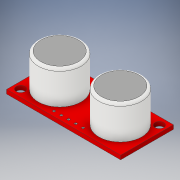
# Autodesk Inventor part: SRF08
Saved by Autodesk Inventor 2018 (Build 220112000, 112)
## iProperties
Created: 2019-03-05
Part Number: SRF08
Material: Generisch
Document SubType Name: Modeling
Designer: RedBots
Density: 1.3582 g/cm^3
Appearance: Vorgabe
Mass: 9 g
Surface Area: 32.6581 cm^2
Volume: 6.62642 cm^3
Author: RedBots
Autodesk Inventor part; units mm, degrees
ref_plane "YZ Plane" through (0, 0, 0) normal (1, 0, 0) x (0, 1, 0)
ref_plane "XZ Plane" through (0, 0, 0) normal (0, 1, 0) x (-1, 0, 0)
ref_plane "XY Plane" through (0, 0, 0) normal (0, 0, 1) x (1, 0, 0)
sketch "Skizze1" plane through (0, 0, 0) normal (0, 0, 1) x (1, 0, 0)
  line L0 (0, 0) -> (43.18, 0)
  line L1 (43.18, 0) -> (43.18, 20)
  line L2 (43.18, 20) -> (0, 20)
  line L3 (0, 20) -> (0, 0)
  circle A0 centre (2.54, 2.761) radius 1.651
  circle A1 centre (40.64, 17.239) radius 1.651
  line L4 (21.59, 20) -> (21.59, 0) construction
  line L5 (2.54, 2.761) -> (40.64, 2.761) construction
  line L6 (40.64, 2.761) -> (40.64, 17.239) construction
  line L7 (40.64, 17.239) -> (2.54, 17.239) construction
  line L8 (2.54, 17.239) -> (2.54, 2.761) construction
  line L9 (0, 10) -> (43.18, 10) construction
  line L10 (21.965, 2.2486) -> (21.215, 2.2486)
  line L11 (21.215, 2.2486) -> (21.215, 1.4986)
  line L12 (21.215, 1.4986) -> (21.965, 1.4986)
  line L13 (21.965, 1.4986) -> (21.965, 2.2486)
  line L14 (24.715, 2.2486) -> (23.965, 2.2486)
  line L15 (24.715, 1.4986) -> (24.715, 2.2486)
  line L16 (23.965, 1.4986) -> (24.715, 1.4986)
  line L17 (23.965, 2.2486) -> (23.965, 1.4986)
  line L18 (27.465, 2.2486) -> (26.715, 2.2486)
  line L19 (27.465, 1.4986) -> (27.465, 2.2486)
  line L20 (26.715, 1.4986) -> (27.465, 1.4986)
  line L21 (26.715, 2.2486) -> (26.715, 1.4986)
  line L22 (19.215, 2.2486) -> (18.465, 2.2486)
  line L23 (19.215, 1.4986) -> (19.215, 2.2486)
  line L24 (18.465, 1.4986) -> (19.215, 1.4986)
  line L25 (18.465, 2.2486) -> (18.465, 1.4986)
  line L26 (21.965, 2.2486) -> (21.215, 2.2486)
  line L27 (21.965, 1.4986) -> (21.965, 2.2486)
  line L28 (21.215, 1.4986) -> (21.965, 1.4986)
  line L29 (21.215, 2.2486) -> (21.215, 1.4986)
  line L30 (24.715, 2.2486) -> (23.965, 2.2486)
  line L31 (24.715, 1.4986) -> (24.715, 2.2486)
  line L32 (23.965, 1.4986) -> (24.715, 1.4986)
  line L33 (23.965, 2.2486) -> (23.965, 1.4986)
  line L34 (16.465, 2.2486) -> (15.715, 2.2486)
  line L35 (16.465, 1.4986) -> (16.465, 2.2486)
  line L36 (15.715, 1.4986) -> (16.465, 1.4986)
  line L37 (15.715, 2.2486) -> (15.715, 1.4986)
  line L38 (19.215, 2.2486) -> (18.465, 2.2486)
  line L39 (19.215, 1.4986) -> (19.215, 2.2486)
  line L40 (18.465, 1.4986) -> (19.215, 1.4986)
  line L41 (18.465, 2.2486) -> (18.465, 1.4986)
  line L42 (21.965, 2.2486) -> (21.215, 2.2486)
  line L43 (21.965, 1.4986) -> (21.965, 2.2486)
  line L44 (21.215, 1.4986) -> (21.965, 1.4986)
  line L45 (21.215, 2.2486) -> (21.215, 1.4986)
  point P0 (21.59, 17.239)
  point P1 (40.64, 10)
  point P2 (21.59, 2.2486)
  point P3 (24.34, 2.2486)
  point P4 (27.09, 2.2486)
  point P5 (18.84, 2.2486)
  point P6 (21.59, 2.2486)
  point P7 (24.34, 2.2486)
  point P8 (16.09, 2.2486)
  point P9 (18.84, 2.2486)
  point P10 (21.59, 2.2486)
  dimension "d0" = 43.18
  dimension "d1" = 20
  dimension "d2" = 3.302
  dimension "d4" = 38.1
  dimension "d5" = 14.478
  dimension "d26" = 1.4986
  dimension "d27" = 0.75
  dimension "d30" = 2.75
  dimension "d33" = 2.75
  constraints: 92 end point, 7 midpoint, 6 parallel, 5 horizontal, 4 perpendicular, 3 point on line, 2 centre point, 1 equal radius, 72 other
  measures "d0" distance of L2.end L1.end
  measures "d1" distance of L1.end L0.end
  measures "d2" diameter of A0
  measures "d4" distance of L6.end L7.end
  measures "d5" distance of L5.end L6.end
  measures "d26" distance between parallel lines of L0 L12
  measures "d27" distance of L10.start L10.end
  measures "d30" distance of L10.start L14.start
  measures "d33" distance of L10.start L22.start
extrude "Extrusion1" add sketch "Skizze1" against normal blind 1.524
sketch "Skizze2" plane through (0, 0, 0) normal (0, 0, 1) x (1, 0, 0)
  circle A0 centre (10.1127, 10) radius 8.128
  circle A1 centre (33.0673, 10) radius 8.128
  line L0 (0, 0) -> (0, 20) construction
  line L1 (0, 10) -> (43.18, 10) construction
  line L2 (43.18, 0) -> (43.18, 20) construction
  line L3 (10.1127, 10) -> (33.0673, 10) construction
  point P0 (21.59, 10)
  dimension "d19" = 16.256
  constraints: 4 end point, 4 midpoint, 2 centre point, 2 point on line, 1 collinear, 1 equal radius
  measures "d19" diameter of A0
extrude "Extrusion2" add sketch "Skizze2" along normal blind 12.7
fillet "Rundung1" radius 1 2 edges at (24.9393, 10, 12.7) (1.9847, 10, 12.7)
sketch "Skizze3" plane through (0, 0, 0) normal (0, 0, 1) x (1, 0, 0)
  line L0 (43.18, 20) -> (0, 20) construction
  line L1 (21.59, 20) -> (21.59, 16.583) construction
  circle A0 centre (21.59, 16.583) radius 2.286
  point P0 (0, 0)
  dimension "d23" = 4.572
  constraints: 2 end point, 1 centre point, 1 coincident, 1 midpoint, 1 vertical
  measures "d23" diameter of A0
extrude "Extrusion3" add sketch "Skizze3" along normal blind 5.5
